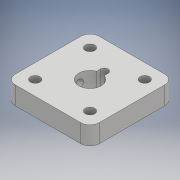
# Autodesk Inventor part: 車輪ハブ3
Saved by Autodesk Inventor 2017 (Build 210142000, 142)
## iProperties
Part Number: 車輪ハブ3
Material: 一般
Document SubType Name: Modeling
Designer: highs
Density: 1 g/cm^3
Appearance: 既定
Author: highs
Autodesk Inventor part; units mm, degrees
ref_plane "YZ Plane" through (0, 0, 0) normal (1, 0, 0) x (0, 1, 0)
ref_plane "XZ Plane" through (0, 0, 0) normal (0, 1, 0) x (-1, 0, 0)
ref_plane "XY Plane" through (0, 0, 0) normal (0, 0, 1) x (1, 0, 0)
sketch "スケッチ1" plane through (0, 0, 0) normal (0, 0, 1) x (1, 0, 0)
  circle A0 centre (0, 0) radius 6.1
  circle A1 centre (0, 0) radius 21.2132 construction
  line L0 (0, 0) -> (15, 15) construction
  line L1 (0, 0) -> (0, 37.5908) construction
  circle A2 centre (15, 15) radius 2.6
  circle A3 centre (-15, 15) radius 2.6
  circle A4 centre (-15, -15) radius 2.6
  circle A5 centre (15, -15) radius 2.6
  line L2 (-15, 15) -> (15, 15) construction
  line L3 (15, 15) -> (15, -15) construction
  line L4 (15, -15) -> (-15, -15) construction
  line L5 (-15, -15) -> (-15, 15) construction
  line L6 (-23, -23) -> (23, -23)
  line L7 (23, -23) -> (23, 23)
  line L8 (23, 23) -> (-23, 23)
  line L9 (-23, 23) -> (-23, -23)
  line L10 (-23, -23) -> (23, 23) construction
  line L11 (23, -23) -> (-23, 23) construction
  circle A6 centre (0, 0) radius 15 construction
  circle A7 centre (-15, 15) radius 5.7791 construction
  dimension "d1" = 12.2
  dimension "d3" = 45
  dimension "d4" = 5.2
  dimension "d7" = 360
  dimension "d11" = 30
  dimension "d12" = 46
  constraints: 24 end point, 8 centre point, 5 coincident, 2 horizontal, 2 midpoint, 2 parallel, 2 perpendicular, 2 point on circle, 1 point on line, 1 tangent, 1 vertical, 9 other
  measures "d1" diameter of A0
  measures "d3" angle of L1 L0
  measures "d4" diameter of A2
  measures "d11" distance of L2.start L2.end
  measures "d12" distance of L8.end L6.start
extrude "押し出し1" add sketch "スケッチ1" along normal blind 10
sketch "スケッチ2" plane through (-23, -23, 0) normal (-1, 0, 0) x (0, 0, 1)
  line L0 (0, 23) -> (10, 23) construction
  line L1 (10, 29.1) -> (10, 16.9) construction
  circle A0 centre (5, 23) radius 2.1
  dimension "d14" = 4.2
  constraints: 2 end point, 2 midpoint, 1 centre point
  measures "d14" diameter of A0
extrude "押し出し2" cut sketch "スケッチ2" against normal up to next
fillet "フィレット2" radius 5 4 edges at (23, -23, 5) (23, 23, 5) (-23, -23, 5) (-23, 23, 5)
sketch "スケッチ3" plane through (0, 0, 10) normal (0, 0, 1) x (1, 0, 0)
  circle A0 centre (0, 0) radius 6.1 projected
  line L0 (-2.1, 5.7271) -> (-2.1, 7.8)
  line L1 (-2.1, 7.8) -> (2.1, 7.8) construction
  line L2 (2.1, 7.8) -> (2.1, 5.7271)
  line L3 (0, 0) -> (0, 23) construction
  line L4 (18, 23) -> (-18, 23) construction
  arc A1 (2.1, 7.8) -> (-2.1, 7.8) centre (0, 7.8) ccw
  line L5 (-2.1, 5.7271) -> (2.1, 5.7271)
  point P0 (0, 6.1)
  dimension "d18" = 2.1
  dimension "d23" = 7.8
  constraints: 10 end point, 5 point on circle, 2 midpoint, 2 perpendicular, 2 point on line, 1 centre point, 1 horizontal, 1 vertical, 1 other
  measures "d18" radius of A1
  measures "d23" distance from line of L1 point (0, 0)
extrude "押し出し3" cut sketch "スケッチ3" against normal blind 10 contours A0 L0 A1 L2
